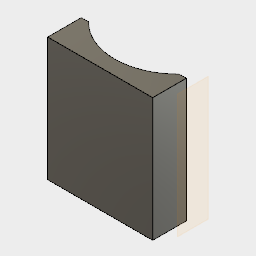
soporte_IMU (Autodesk Fusion 360 design; units mm, degrees)
Autodesk Fusion 360 part; units mm, degrees
sketch "Sketch1" plane through (0, 0, 0) normal (0, 1, 0) x (1, 0, 0)
  circle A0 centre (0, 0) radius 20
  dimension "d1" = 40
  measures "d1" diameter of A0
extrude "Extrude1" add sketch "Sketch1" along normal blind 140
sketch "Sketch2" plane through (0, 140, 0) normal (0, 1, 0) x (-1, 0, 0)
  circle A0 centre (0, 0) radius 20
  circle A1 centre (0, 0) radius 17
  dimension "d4" = 34
  measures "d4" diameter of A1
extrude "Extrude2" add sketch "Sketch2" along normal blind 20 contours A1
sketch "Sketch3" plane through (0, 0, 0) normal (1, 0, 0) x (0, 0, -1)
sketch "Sketch4" plane through (0, 0, 0) normal (0, -1, 0) x (1, 0, 0)
  circle A0 centre (0, 0) radius 20
  line L0 (0, 20) -> (-20, 20)
  line L1 (-20, 20) -> (-20, 10)
  line L2 (-20, 10) -> (20, 10)
  line L3 (20, 10) -> (20, 20)
  line L4 (20, 20) -> (0, 20)
extrude "Extrude3" add sketch "Sketch4" against normal blind 40 contours A0 L2 L3 L4 | A0 L0 L1 L2
sketch "Sketch5" plane through (20, 0, 0) normal (1, 0, 0) x (0, 0, -1)
  line L0 (-20, 0) -> (-10, 0)
  line L1 (-10, 0) -> (-10, 40)
  line L2 (-10, 40) -> (-20, 40)
  line L3 (-20, 40) -> (-20, 0)
sketch "Sketch6" plane through (0, 0, 0) normal (0, 1, 0) x (1, 0, 0)
extrude "Extrude4" add 1 faces at (0, 13.3333, 20) along direction (0, 0, 1) blind 5
sketch "Sketch7" plane through (0, 0, 0) normal (0, 1, 0) x (1, 0, 0)
  circle A0 centre (0, 0) radius 20.3
  dimension "d15" = 40.6
  measures "d15" diameter of A0
extrude "Extrude5" cut sketch "Sketch7" along normal blind 165
extrude "Extrude6" cut 1 faces at (-20, 13.3333, 20) along direction (1, 0, 0) blind 3
extrude "Extrude7" cut 1 faces at (20, 13.3333, 20) along direction (-1, 0, 0) blind 3
sketch "Sketch8" plane through (0, 0, 0) normal (1, 0, 0) x (0, 0, -1)
  line L0 (-11.0946, 40) -> (-14.0946, 40)
  line L1 (-14.0946, 40) -> (-14.0946, -0.0914)
  line L2 (-14.0946, -0.0914) -> (-11.0946, -0.0914)
  line L3 (-11.0946, -0.0914) -> (-11.0946, 40)
  point P0 (-11.0946, 40)
  dimension "d22" = 3
  measures "d22" distance of P0 L0.end
extrude "Extrude8" cut sketch "Sketch8" along normal blind 20 and the other way blind 20
